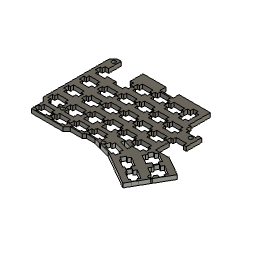
open-backplate-heatset-insert (Autodesk Fusion 360 design; units mm, degrees)
Autodesk Fusion 360 part; units mm, degrees
sketch "Sketch1" plane through (0, 0, 0) normal (0, 0, 1) x (1, 0, 0)
  line L0 (38.6885, 37.314) -> (36.2135, 37.314)
  line L1 (36.2135, 37.314) -> (36.2135, 63.246)
  line L2 (36.2135, 63.246) -> (-1.4615, 63.246)
  line L3 (-1.4615, 63.246) -> (-1.4615, 56.246)
  line L4 (-1.4615, 56.246) -> (-17.4615, 56.246)
  line L5 (-17.4615, 56.246) -> (-17.4615, 63.246)
  line L6 (-17.4615, 63.246) -> (-45.1095, 63.246)
  line L7 (-45.1095, 63.246) -> (-45.1095, 47.839)
  line L8 (-45.1095, 47.839) -> (-41.2315, 47.839)
  line L9 (-41.2315, 47.839) -> (-41.2315, 44.299)
  line L10 (-41.2315, 44.299) -> (-38.5615, 44.299)
  line L11 (-38.5615, 44.299) -> (-38.5615, 38.759)
  line L12 (-38.5615, 38.759) -> (-42.0615, 38.759)
  line L13 (-42.0615, 38.759) -> (-42.0615, 35.339)
  line L14 (-42.0615, 35.339) -> (-53.0615, 35.339)
  line L15 (-53.0615, 35.339) -> (-53.0615, 38.759)
  line L16 (-53.0615, 38.759) -> (-63.6515, 38.759)
  line L17 (-63.6515, 38.759) -> (-63.6515, 35.339)
  line L18 (-63.6515, 35.339) -> (-74.6515, 35.339)
  line L19 (-74.6515, 35.339) -> (-74.6515, 38.759)
  line L20 (-74.6515, 38.759) -> (-78.1515, 38.759)
  line L21 (-78.1515, 38.759) -> (-78.1515, 44.299)
  line L22 (-78.1515, 44.299) -> (-75.4815, 44.299)
  line L23 (-75.4815, 44.299) -> (-75.4815, 47.839)
  line L24 (-75.4815, 47.839) -> (-71.3495, 47.839)
  line L25 (-71.3495, 47.839) -> (-71.3495, 63.246)
  line L26 (-71.3495, 63.246) -> (-76.0095, 63.246)
  line L27 (-76.0095, 63.246) -> (-81.0895, 58.166)
  line L28 (-81.0895, 58.166) -> (-81.0895, -21.336)
  line L29 (-81.0895, -21.336) -> (-76.2635, -26.162)
  line L30 (-76.2635, -26.162) -> (-76.2635, -40.386)
  line L31 (-76.2635, -40.386) -> (-38.1635, -40.386)
  line L32 (-38.1635, -40.386) -> (-33.8455, -36.068)
  line L33 (-33.8455, -36.068) -> (-19.1135, -36.068)
  line L34 (-19.1135, -36.068) -> (-16.5735, -33.528)
  line L35 (-16.5735, -33.528) -> (-6.4135, -33.528)
  line L36 (-6.4135, -33.528) -> (1.2965, -35.5781)
  line L37 (1.2965, -35.5781) -> (0.5808, -35.056)
  line L38 (0.5808, -35.056) -> (0.019, -34.371)
  line L39 (0.019, -34.371) -> (-0.3528, -33.5668)
  line L40 (-0.3528, -33.5668) -> (-0.5107, -32.6951)
  line L41 (-0.5107, -32.6951) -> (-0.4447, -31.8116)
  line L42 (-0.4447, -31.8116) -> (-0.159, -30.973)
  line L43 (-0.159, -30.973) -> (0.3281, -30.233)
  line L44 (0.3281, -30.233) -> (0.9854, -29.6391)
  line L45 (0.9854, -29.6391) -> (1.7708, -29.2292)
  line L46 (1.7708, -29.2292) -> (2.634, -29.0296)
  line L47 (2.634, -29.0296) -> (3.5196, -29.0532)
  line L48 (3.5196, -29.0532) -> (4.3709, -29.2983)
  line L49 (4.3709, -29.2983) -> (5.1334, -29.7494)
  line L50 (5.1334, -29.7494) -> (5.7582, -30.3775)
  line L51 (5.7582, -30.3775) -> (6.2053, -31.1423)
  line L52 (6.2053, -31.1423) -> (6.976, -28.2662)
  line L53 (6.976, -28.2662) -> (9.555, -28.9572)
  line L54 (9.555, -28.9572) -> (10.4712, -25.5379)
  line L55 (10.4712, -25.5379) -> (22.6999, -28.8145)
  line L56 (22.6999, -28.8145) -> (21.7836, -32.2339)
  line L57 (21.7836, -32.2339) -> (24.3627, -32.9249)
  line L58 (24.3627, -32.9249) -> (22.9288, -38.2762)
  line L59 (22.9288, -38.2762) -> (19.5481, -37.3703)
  line L60 (19.5481, -37.3703) -> (19.1145, -38.9882)
  line L61 (19.1145, -38.9882) -> (8.4894, -36.1412)
  line L62 (8.4894, -36.1412) -> (8.9229, -34.5233)
  line L63 (8.9229, -34.5233) -> (6.2374, -33.8037)
  line L64 (6.2374, -33.8037) -> (5.8334, -34.5452)
  line L65 (5.8334, -34.5452) -> (5.2635, -35.1684)
  line L66 (5.2635, -35.1684) -> (4.5609, -35.6369)
  line L67 (4.5609, -35.6369) -> (3.7666, -35.9235)
  line L68 (3.7666, -35.9235) -> (2.9267, -36.0115)
  line L69 (2.9267, -36.0115) -> (15.5575, -39.37)
  line L70 (15.5575, -39.37) -> (56.9595, -63.246)
  line L71 (56.9595, -63.246) -> (57.0865, -63.246)
  line L72 (57.0865, -63.246) -> (69.3649, -41.9374)
  line L73 (69.3649, -41.9374) -> (68.7057, -42.5189)
  line L74 (68.7057, -42.5189) -> (67.9224, -42.9177)
  line L75 (67.9224, -42.9177) -> (67.0644, -43.1088)
  line L76 (67.0644, -43.1088) -> (66.1858, -43.0801)
  line L77 (66.1858, -43.0801) -> (65.3421, -42.8334)
  line L78 (65.3421, -42.8334) -> (64.5865, -42.3843)
  line L79 (64.5865, -42.3843) -> (63.9667, -41.761)
  line L80 (63.9667, -41.761) -> (63.5216, -41.003)
  line L81 (63.5216, -41.003) -> (63.2795, -40.158)
  line L82 (63.2795, -40.158) -> (63.2555, -39.2793)
  line L83 (63.2555, -39.2793) -> (63.4512, -38.4224)
  line L84 (63.4512, -38.4224) -> (63.8543, -37.6412)
  line L85 (63.8543, -37.6412) -> (64.4393, -36.9851)
  line L86 (64.4393, -36.9851) -> (56.2282, -32.2241)
  line L87 (56.2282, -32.2241) -> (57.7331, -29.6288)
  line L88 (57.7331, -29.6288) -> (58.953, -27.5158)
  line L89 (58.953, -27.5158) -> (56.9243, -26.3445)
  line L90 (56.9243, -26.3445) -> (59.6943, -21.5467)
  line L91 (59.6943, -21.5467) -> (62.0066, -22.8817)
  line L92 (62.0066, -22.8817) -> (63.7766, -19.8159)
  line L93 (63.7766, -19.8159) -> (74.7404, -26.1459)
  line L94 (74.7404, -26.1459) -> (72.9704, -29.2117)
  line L95 (72.9704, -29.2117) -> (75.2827, -30.5467)
  line L96 (75.2827, -30.5467) -> (72.5127, -35.3445)
  line L97 (72.5127, -35.3445) -> (69.7783, -33.7657)
  line L98 (69.7783, -33.7657) -> (68.5467, -35.8989)
  line L99 (68.5467, -35.8989) -> (68.2253, -36.4557)
  line L100 (68.2253, -36.4557) -> (68.9421, -36.9048)
  line L101 (68.9421, -36.9048) -> (69.5309, -37.5139)
  line L102 (69.5309, -37.5139) -> (69.956, -38.2466)
  line L103 (69.956, -38.2466) -> (70.1927, -39.0599)
  line L104 (70.1927, -39.0599) -> (70.2271, -39.9063)
  line L105 (70.2271, -39.9063) -> (70.0571, -40.7362)
  line L106 (70.0571, -40.7362) -> (81.0895, -21.59)
  line L107 (81.0895, -21.59) -> (57.2135, -7.874)
  line L108 (57.2135, -7.874) -> (57.2135, -8.776)
  line L109 (57.2135, -8.776) -> (42.1885, -8.776)
  line L110 (42.1885, -8.776) -> (42.1885, 7.644)
  line L111 (42.1885, 7.644) -> (38.6885, 7.644)
  line L112 (38.6885, 7.644) -> (38.6885, 13.184)
  line L113 (38.6885, 13.184) -> (41.3585, 13.184)
  line L114 (41.3585, 13.184) -> (41.3585, 16.724)
  line L115 (41.3585, 16.724) -> (54.0185, 16.724)
  line L116 (54.0185, 16.724) -> (54.0185, 13.184)
  line L117 (54.0185, 13.184) -> (57.2135, 13.184)
  line L118 (57.2135, 13.184) -> (57.2135, 31.774)
  line L119 (57.2135, 31.774) -> (53.1885, 31.774)
  line L120 (53.1885, 31.774) -> (53.1885, 28.354)
  line L121 (53.1885, 28.354) -> (52.1361, 28.354)
  line L122 (52.1361, 28.354) -> (52.9138, 27.8863)
  line L123 (52.9138, 27.8863) -> (53.5451, 27.2344)
  line L124 (53.5451, 27.2344) -> (53.9877, 26.4421)
  line L125 (53.9877, 26.4421) -> (54.2116, 25.5627)
  line L126 (54.2116, 25.5627) -> (54.2019, 24.6552)
  line L127 (54.2019, 24.6552) -> (53.9593, 23.7808)
  line L128 (53.9593, 23.7808) -> (53.4999, 22.9981)
  line L129 (53.4999, 22.9981) -> (52.8548, 22.3598)
  line L130 (52.8548, 22.3598) -> (52.0673, 21.9089)
  line L131 (52.0673, 21.9089) -> (51.1903, 21.6755)
  line L132 (51.1903, 21.6755) -> (50.2828, 21.6755)
  line L133 (50.2828, 21.6755) -> (49.4057, 21.9089)
  line L134 (49.4057, 21.9089) -> (48.6182, 22.3598)
  line L135 (48.6182, 22.3598) -> (47.9731, 22.9981)
  line L136 (47.9731, 22.9981) -> (47.5137, 23.7808)
  line L137 (47.5137, 23.7808) -> (47.2711, 24.6552)
  line L138 (47.2711, 24.6552) -> (47.2614, 25.5627)
  line L139 (47.2614, 25.5627) -> (47.4853, 26.4421)
  line L140 (47.4853, 26.4421) -> (47.9279, 27.2344)
  line L141 (47.9279, 27.2344) -> (48.5592, 27.8863)
  line L142 (48.5592, 27.8863) -> (49.337, 28.354)
  line L143 (49.337, 28.354) -> (42.1885, 28.354)
  line L144 (42.1885, 28.354) -> (42.1885, 31.774)
  line L145 (42.1885, 31.774) -> (38.6885, 31.774)
  line L146 (38.6885, 31.774) -> (38.6885, 37.314)
  line L147 (-71.8668, 59.0719) -> (-71.7475, 58.166)
  line L148 (-71.7475, 58.166) -> (-71.8668, 57.2601)
  line L149 (-71.8668, 57.2601) -> (-72.2164, 56.416)
  line L150 (-72.2164, 56.416) -> (-72.7726, 55.6911)
  line L151 (-72.7726, 55.6911) -> (-73.4975, 55.1349)
  line L152 (-73.4975, 55.1349) -> (-74.3416, 54.7853)
  line L153 (-74.3416, 54.7853) -> (-75.2475, 54.666)
  line L154 (-75.2475, 54.666) -> (-76.1534, 54.7853)
  line L155 (-76.1534, 54.7853) -> (-76.9975, 55.1349)
  line L156 (-76.9975, 55.1349) -> (-77.7224, 55.6911)
  line L157 (-77.7224, 55.6911) -> (-78.2786, 56.416)
  line L158 (-78.2786, 56.416) -> (-78.6282, 57.2601)
  line L159 (-78.6282, 57.2601) -> (-78.7475, 58.166)
  line L160 (-78.7475, 58.166) -> (-78.6282, 59.0719)
  line L161 (-78.6282, 59.0719) -> (-78.2786, 59.916)
  line L162 (-78.2786, 59.916) -> (-77.7224, 60.6409)
  line L163 (-77.7224, 60.6409) -> (-76.9975, 61.1971)
  line L164 (-76.9975, 61.1971) -> (-76.1534, 61.5467)
  line L165 (-76.1534, 61.5467) -> (-75.2475, 61.666)
  line L166 (-75.2475, 61.666) -> (-74.3416, 61.5467)
  line L167 (-74.3416, 61.5467) -> (-73.4975, 61.1971)
  line L168 (-73.4975, 61.1971) -> (-72.7726, 60.6409)
  line L169 (-72.7726, 60.6409) -> (-72.2164, 59.916)
  line L170 (-72.2164, 59.916) -> (-71.8668, 59.0719)
  line L171 (-53.0615, -18.4285) -> (-55.7119, -18.4285)
  line L172 (-55.7119, -18.4285) -> (-54.9733, -18.9008)
  line L173 (-54.9733, -18.9008) -> (-54.3753, -19.5419)
  line L174 (-54.3753, -19.5419) -> (-53.9554, -20.3114)
  line L175 (-53.9554, -20.3114) -> (-53.7399, -21.1611)
  line L176 (-53.7399, -21.1611) -> (-53.7423, -22.0378)
  line L177 (-53.7423, -22.0378) -> (-53.9624, -22.8863)
  line L178 (-53.9624, -22.8863) -> (-54.3865, -23.6536)
  line L179 (-54.3865, -23.6536) -> (-54.988, -24.2913)
  line L180 (-54.988, -24.2913) -> (-55.7291, -24.7596)
  line L181 (-55.7291, -24.7596) -> (-56.5633, -25.0291)
  line L182 (-56.5633, -25.0291) -> (-57.4383, -25.0828)
  line L183 (-57.4383, -25.0828) -> (-58.2992, -24.9174)
  line L184 (-58.2992, -24.9174) -> (-59.092, -24.5432)
  line L185 (-59.092, -24.5432) -> (-59.7669, -23.9837)
  line L186 (-59.7669, -23.9837) -> (-60.2817, -23.2741)
  line L187 (-60.2817, -23.2741) -> (-60.6039, -22.4589)
  line L188 (-60.6039, -22.4589) -> (-60.7135, -21.5891)
  line L189 (-60.7135, -21.5891) -> (-60.6035, -20.7194)
  line L190 (-60.6035, -20.7194) -> (-60.2808, -19.9043)
  line L191 (-60.2808, -19.9043) -> (-59.7657, -19.1949)
  line L192 (-59.7657, -19.1949) -> (-59.0904, -18.6358)
  line L193 (-59.0904, -18.6358) -> (-58.2975, -18.2621)
  line L194 (-58.2975, -18.2621) -> (-57.4365, -18.0971)
  line L195 (-57.4365, -18.0971) -> (-56.5615, -18.1513)
  line L196 (-56.5615, -18.1513) -> (-56.5615, -12.8885)
  line L197 (-56.5615, -12.8885) -> (-53.8915, -12.8885)
  line L198 (-53.8915, -12.8885) -> (-53.8915, -9.3485)
  line L199 (-53.8915, -9.3485) -> (-41.2315, -9.3485)
  line L200 (-41.2315, -9.3485) -> (-41.2315, -12.8885)
  line L201 (-41.2315, -12.8885) -> (-38.5615, -12.8885)
  line L202 (-38.5615, -12.8885) -> (-38.5615, -18.4285)
  line L203 (-38.5615, -18.4285) -> (-42.0615, -18.4285)
  line L204 (-42.0615, -18.4285) -> (-42.0615, -23.852)
  line L205 (-42.0615, -23.852) -> (-53.0615, -23.852)
  line L206 (-53.0615, -23.852) -> (-53.0615, -18.4285)
  line L207 (-53.0615, -37.491) -> (-53.0615, -39.166)
  line L208 (-53.0615, -39.166) -> (-42.0615, -39.166)
  line L209 (-42.0615, -39.166) -> (-42.0615, -37.491)
  line L210 (-42.0615, -37.491) -> (-38.5615, -37.491)
  line L211 (-38.5615, -37.491) -> (-38.5615, -31.951)
  line L212 (-38.5615, -31.951) -> (-41.2315, -31.951)
  line L213 (-41.2315, -31.951) -> (-41.2315, -28.411)
  line L214 (-41.2315, -28.411) -> (-53.8915, -28.411)
  line L215 (-53.8915, -28.411) -> (-53.8915, -31.951)
  line L216 (-53.8915, -31.951) -> (-56.5615, -31.951)
  line L217 (-56.5615, -31.951) -> (-56.5615, -37.491)
  line L218 (-56.5615, -37.491) -> (-53.0615, -37.491)
  line L219 (-14.9615, -30.506) -> (-14.9615, -32.181)
  line L220 (-14.9615, -32.181) -> (-3.9615, -32.181)
  line L221 (-3.9615, -32.181) -> (-3.9615, -30.506)
  line L222 (-3.9615, -30.506) -> (-0.4615, -30.506)
  line L223 (-0.4615, -30.506) -> (-0.4615, -24.966)
  line L224 (-0.4615, -24.966) -> (-3.1315, -24.966)
  line L225 (-3.1315, -24.966) -> (-3.1315, -21.426)
  line L226 (-3.1315, -21.426) -> (-15.7915, -21.426)
  line L227 (-15.7915, -21.426) -> (-15.7915, -24.966)
  line L228 (-15.7915, -24.966) -> (-18.4615, -24.966)
  line L229 (-18.4615, -24.966) -> (-18.4615, -30.506)
  line L230 (-18.4615, -30.506) -> (-14.9615, -30.506)
  line L231 (47.8904, -49.0495) -> (47.0529, -50.5)
  line L232 (47.0529, -50.5) -> (56.5791, -56)
  line L233 (56.5791, -56) -> (57.4166, -54.5495)
  line L234 (57.4166, -54.5495) -> (60.4477, -56.2995)
  line L235 (60.4477, -56.2995) -> (63.2177, -51.5017)
  line L236 (63.2177, -51.5017) -> (60.9054, -50.1667)
  line L237 (60.9054, -50.1667) -> (62.6754, -47.1009)
  line L238 (62.6754, -47.1009) -> (51.7116, -40.7709)
  line L239 (51.7116, -40.7709) -> (49.9416, -43.8367)
  line L240 (49.9416, -43.8367) -> (47.6293, -42.5017)
  line L241 (47.6293, -42.5017) -> (44.8593, -47.2995)
  line L242 (44.8593, -47.2995) -> (47.8904, -49.0495)
  line L243 (31.3804, -39.5245) -> (30.5429, -40.9751)
  line L244 (30.5429, -40.9751) -> (40.0691, -46.4751)
  line L245 (40.0691, -46.4751) -> (40.9066, -45.0245)
  line L246 (40.9066, -45.0245) -> (43.9377, -46.7745)
  line L247 (43.9377, -46.7745) -> (46.7077, -41.9767)
  line L248 (46.7077, -41.9767) -> (44.3954, -40.6417)
  line L249 (44.3954, -40.6417) -> (46.1654, -37.5759)
  line L250 (46.1654, -37.5759) -> (35.2016, -31.2459)
  line L251 (35.2016, -31.2459) -> (33.4316, -34.3117)
  line L252 (33.4316, -34.3117) -> (31.1193, -32.9767)
  line L253 (31.1193, -32.9767) -> (28.3493, -37.7745)
  line L254 (28.3493, -37.7745) -> (31.3804, -39.5245)
  line L255 (-72.1115, -37.441) -> (-72.1115, -39.1189)
  line L256 (-72.1115, -39.1189) -> (-61.1115, -39.1189)
  line L257 (-61.1115, -39.1189) -> (-61.1115, -37.441)
  line L258 (-61.1115, -37.441) -> (-57.6115, -37.441)
  line L259 (-57.6115, -37.441) -> (-57.6115, -31.901)
  line L260 (-57.6115, -31.901) -> (-60.2815, -31.901)
  line L261 (-60.2815, -31.901) -> (-60.2815, -28.361)
  line L262 (-60.2815, -28.361) -> (-72.9415, -28.361)
  line L263 (-72.9415, -28.361) -> (-72.9415, -31.901)
  line L264 (-72.9415, -31.901) -> (-75.6115, -31.901)
  line L265 (-75.6115, -31.901) -> (-75.6115, -37.441)
  line L266 (-75.6115, -37.441) -> (-72.1115, -37.441)
  line L267 (-0.4615, 7.619) -> (-0.4615, 13.159)
  line L268 (-0.4615, 13.159) -> (-3.1315, 13.159)
  line L269 (-3.1315, 13.159) -> (-3.1315, 16.699)
  line L270 (-3.1315, 16.699) -> (-15.7915, 16.699)
  line L271 (-15.7915, 16.699) -> (-15.7915, 13.159)
  line L272 (-15.7915, 13.159) -> (-18.4615, 13.159)
  line L273 (-18.4615, 13.159) -> (-18.4615, 7.619)
  line L274 (-18.4615, 7.619) -> (-14.9615, 7.619)
  line L275 (-14.9615, 7.619) -> (-14.9615, 4.199)
  line L276 (-14.9615, 4.199) -> (-3.9615, 4.199)
  line L277 (-3.9615, 4.199) -> (-3.9615, 7.619)
  line L278 (-3.9615, 7.619) -> (-0.4615, 7.619)
  line L279 (-34.0115, -33.046) -> (-34.0115, -34.721)
  line L280 (-34.0115, -34.721) -> (-23.0115, -34.721)
  line L281 (-23.0115, -34.721) -> (-23.0115, -33.046)
  line L282 (-23.0115, -33.046) -> (-19.5115, -33.046)
  line L283 (-19.5115, -33.046) -> (-19.5115, -27.506)
  line L284 (-19.5115, -27.506) -> (-22.1815, -27.506)
  line L285 (-22.1815, -27.506) -> (-22.1815, -23.966)
  line L286 (-22.1815, -23.966) -> (-34.8415, -23.966)
  line L287 (-34.8415, -23.966) -> (-34.8415, -27.506)
  line L288 (-34.8415, -27.506) -> (-37.5115, -27.506)
  line L289 (-37.5115, -27.506) -> (-37.5115, -33.046)
  line L290 (-37.5115, -33.046) -> (-34.0115, -33.046)
  line L291 (-19.5115, 43.204) -> (-19.5115, 48.744)
  line L292 (-19.5115, 48.744) -> (-22.1815, 48.744)
  line L293 (-22.1815, 48.744) -> (-22.1815, 52.284)
  line L294 (-22.1815, 52.284) -> (-34.8415, 52.284)
  line L295 (-34.8415, 52.284) -> (-34.8415, 48.744)
  line L296 (-34.8415, 48.744) -> (-37.5115, 48.744)
  line L297 (-37.5115, 48.744) -> (-37.5115, 43.204)
  line L298 (-37.5115, 43.204) -> (-34.0115, 43.204)
  line L299 (-34.0115, 43.204) -> (-34.0115, 39.784)
  line L300 (-34.0115, 39.784) -> (-23.0115, 39.784)
  line L301 (-23.0115, 39.784) -> (-23.0115, 43.204)
  line L302 (-23.0115, 43.204) -> (-19.5115, 43.204)
  line L303 (15.9185, -8.256) -> (15.9185, -4.716)
  line L304 (15.9185, -4.716) -> (3.2585, -4.716)
  line L305 (3.2585, -4.716) -> (3.2585, -8.256)
  line L306 (3.2585, -8.256) -> (0.5885, -8.256)
  line L307 (0.5885, -8.256) -> (0.5885, -13.796)
  line L308 (0.5885, -13.796) -> (4.0885, -13.796)
  line L309 (4.0885, -13.796) -> (4.0885, -17.216)
  line L310 (4.0885, -17.216) -> (15.0885, -17.216)
  line L311 (15.0885, -17.216) -> (15.0885, -13.796)
  line L312 (15.0885, -13.796) -> (18.5885, -13.796)
  line L313 (18.5885, -13.796) -> (18.5885, -8.256)
  line L314 (18.5885, -8.256) -> (15.9185, -8.256)
  line L315 (-34.0115, -13.9835) -> (-34.0115, -19.534)
  line L316 (-34.0115, -19.534) -> (-23.0115, -19.534)
  line L317 (-23.0115, -19.534) -> (-23.0115, -13.9835)
  line L318 (-23.0115, -13.9835) -> (-19.5115, -13.9835)
  line L319 (-19.5115, -13.9835) -> (-19.5115, -8.4435)
  line L320 (-19.5115, -8.4435) -> (-22.1815, -8.4435)
  line L321 (-22.1815, -8.4435) -> (-22.1815, -4.9035)
  line L322 (-22.1815, -4.9035) -> (-34.8415, -4.9035)
  line L323 (-34.8415, -4.9035) -> (-34.8415, -8.4435)
  line L324 (-34.8415, -8.4435) -> (-37.5115, -8.4435)
  line L325 (-37.5115, -8.4435) -> (-37.5115, -13.9835)
  line L326 (-37.5115, -13.9835) -> (-34.0115, -13.9835)
  line L327 (58.7727, -21.0217) -> (56.4604, -19.6867)
  line L328 (56.4604, -19.6867) -> (58.2304, -16.6209)
  line L329 (58.2304, -16.6209) -> (47.2666, -10.2909)
  line L330 (47.2666, -10.2909) -> (45.4966, -13.3567)
  line L331 (45.4966, -13.3567) -> (43.1843, -12.0217)
  line L332 (43.1843, -12.0217) -> (40.4143, -16.8195)
  line L333 (40.4143, -16.8195) -> (42.443, -17.9908)
  line L334 (42.443, -17.9908) -> (41.2231, -20.1038)
  line L335 (41.2231, -20.1038) -> (39.7182, -22.6991)
  line L336 (39.7182, -22.6991) -> (50.5319, -28.9692)
  line L337 (50.5319, -28.9692) -> (52.0367, -26.3739)
  line L338 (52.0367, -26.3739) -> (53.2683, -24.2408)
  line L339 (53.2683, -24.2408) -> (56.0027, -25.8195)
  line L340 (56.0027, -25.8195) -> (58.7727, -21.0217)
  line L341 (-19.5115, 10.619) -> (-22.1815, 10.619)
  line L342 (-22.1815, 10.619) -> (-22.1815, 14.159)
  line L343 (-22.1815, 14.159) -> (-34.8415, 14.159)
  line L344 (-34.8415, 14.159) -> (-34.8415, 10.619)
  line L345 (-34.8415, 10.619) -> (-37.5115, 10.619)
  line L346 (-37.5115, 10.619) -> (-37.5115, 5.079)
  line L347 (-37.5115, 5.079) -> (-34.0115, 5.079)
  line L348 (-34.0115, 5.079) -> (-34.0115, 1.659)
  line L349 (-34.0115, 1.659) -> (-23.0115, 1.659)
  line L350 (-23.0115, 1.659) -> (-23.0115, 5.079)
  line L351 (-23.0115, 5.079) -> (-19.5115, 5.079)
  line L352 (-19.5115, 5.079) -> (-19.5115, 10.619)
  line L353 (15.9185, 10.744) -> (15.9185, 14.284)
  line L354 (15.9185, 14.284) -> (3.2585, 14.284)
  line L355 (3.2585, 14.284) -> (3.2585, 10.744)
  line L356 (3.2585, 10.744) -> (0.5885, 10.744)
  line L357 (0.5885, 10.744) -> (0.5885, 5.204)
  line L358 (0.5885, 5.204) -> (4.0885, 5.204)
  line L359 (4.0885, 5.204) -> (4.0885, 1.784)
  line L360 (4.0885, 1.784) -> (15.0885, 1.784)
  line L361 (15.0885, 1.784) -> (15.0885, 5.204)
  line L362 (15.0885, 5.204) -> (18.5885, 5.204)
  line L363 (18.5885, 5.204) -> (18.5885, 10.744)
  line L364 (18.5885, 10.744) -> (15.9185, 10.744)
  line L365 (22.0585, 38.879) -> (27.5985, 38.879)
  line L366 (27.5985, 38.879) -> (27.5985, 41.549)
  line L367 (27.5985, 41.549) -> (31.1385, 41.549)
  line L368 (31.1385, 41.549) -> (31.1385, 54.209)
  line L369 (31.1385, 54.209) -> (27.5985, 54.209)
  line L370 (27.5985, 54.209) -> (27.5985, 56.879)
  line L371 (27.5985, 56.879) -> (22.0585, 56.879)
  line L372 (22.0585, 56.879) -> (22.0585, 53.379)
  line L373 (22.0585, 53.379) -> (18.6385, 53.379)
  line L374 (18.6385, 53.379) -> (18.6385, 42.379)
  line L375 (18.6385, 42.379) -> (22.0585, 42.379)
  line L376 (22.0585, 42.379) -> (22.0585, 38.879)
  line L377 (23.1385, 22.249) -> (23.1385, 18.829)
  line L378 (23.1385, 18.829) -> (34.1385, 18.829)
  line L379 (34.1385, 18.829) -> (34.1385, 22.249)
  line L380 (34.1385, 22.249) -> (37.6385, 22.249)
  line L381 (37.6385, 22.249) -> (37.6385, 27.789)
  line L382 (37.6385, 27.789) -> (34.9685, 27.789)
  line L383 (34.9685, 27.789) -> (34.9685, 31.329)
  line L384 (34.9685, 31.329) -> (22.3085, 31.329)
  line L385 (22.3085, 31.329) -> (22.3085, 27.789)
  line L386 (22.3085, 27.789) -> (19.6385, 27.789)
  line L387 (19.6385, 27.789) -> (19.6385, 22.249)
  line L388 (19.6385, 22.249) -> (23.1385, 22.249)
  line L389 (-0.4615, 26.6815) -> (-0.4615, 32.2215)
  line L390 (-0.4615, 32.2215) -> (-3.1315, 32.2215)
  line L391 (-3.1315, 32.2215) -> (-3.1315, 35.7615)
  line L392 (-3.1315, 35.7615) -> (-15.7915, 35.7615)
  line L393 (-15.7915, 35.7615) -> (-15.7915, 32.2215)
  line L394 (-15.7915, 32.2215) -> (-18.4615, 32.2215)
  line L395 (-18.4615, 32.2215) -> (-18.4615, 26.6815)
  line L396 (-18.4615, 26.6815) -> (-14.9615, 26.6815)
  line L397 (-14.9615, 26.6815) -> (-14.9615, 23.2615)
  line L398 (-14.9615, 23.2615) -> (-3.9615, 23.2615)
  line L399 (-3.9615, 23.2615) -> (-3.9615, 26.6815)
  line L400 (-3.9615, 26.6815) -> (-0.4615, 26.6815)
  line L401 (-19.5115, 29.6815) -> (-22.1815, 29.6815)
  line L402 (-22.1815, 29.6815) -> (-22.1815, 33.2215)
  line L403 (-22.1815, 33.2215) -> (-34.8415, 33.2215)
  line L404 (-34.8415, 33.2215) -> (-34.8415, 29.6815)
  line L405 (-34.8415, 29.6815) -> (-37.5115, 29.6815)
  line L406 (-37.5115, 29.6815) -> (-37.5115, 24.1415)
  line L407 (-37.5115, 24.1415) -> (-34.0115, 24.1415)
  line L408 (-34.0115, 24.1415) -> (-34.0115, 20.7215)
  line L409 (-34.0115, 20.7215) -> (-23.0115, 20.7215)
  line L410 (-23.0115, 20.7215) -> (-23.0115, 24.1415)
  line L411 (-23.0115, 24.1415) -> (-19.5115, 24.1415)
  line L412 (-19.5115, 24.1415) -> (-19.5115, 29.6815)
  line L413 (-60.1515, 25.2157) -> (-62.8215, 25.2157)
  line L414 (-62.8215, 25.2157) -> (-62.8215, 28.7557)
  line L415 (-62.8215, 28.7557) -> (-75.4815, 28.7557)
  line L416 (-75.4815, 28.7557) -> (-75.4815, 25.2157)
  line L417 (-75.4815, 25.2157) -> (-78.1515, 25.2157)
  line L418 (-78.1515, 25.2157) -> (-78.1515, 19.6757)
  line L419 (-78.1515, 19.6757) -> (-74.6515, 19.6757)
  line L420 (-74.6515, 19.6757) -> (-74.6515, 16.2557)
  line L421 (-74.6515, 16.2557) -> (-63.6515, 16.2557)
  line L422 (-63.6515, 16.2557) -> (-63.6515, 19.6757)
  line L423 (-63.6515, 19.6757) -> (-60.1515, 19.6757)
  line L424 (-60.1515, 19.6757) -> (-60.1515, 25.2157)
  line L425 (15.9185, 29.744) -> (15.9185, 33.284)
  line L426 (15.9185, 33.284) -> (3.2585, 33.284)
  line L427 (3.2585, 33.284) -> (3.2585, 29.744)
  line L428 (3.2585, 29.744) -> (0.5885, 29.744)
  line L429 (0.5885, 29.744) -> (0.5885, 24.204)
  line L430 (0.5885, 24.204) -> (4.0885, 24.204)
  line L431 (4.0885, 24.204) -> (4.0885, 20.784)
  line L432 (4.0885, 20.784) -> (15.0885, 20.784)
  line L433 (15.0885, 20.784) -> (15.0885, 24.204)
  line L434 (15.0885, 24.204) -> (18.5885, 24.204)
  line L435 (18.5885, 24.204) -> (18.5885, 29.744)
  line L436 (18.5885, 29.744) -> (15.9185, 29.744)
  line L437 (18.5885, 48.744) -> (15.9185, 48.744)
  line L438 (15.9185, 48.744) -> (15.9185, 52.284)
  line L439 (15.9185, 52.284) -> (3.2585, 52.284)
  line L440 (3.2585, 52.284) -> (3.2585, 48.744)
  line L441 (3.2585, 48.744) -> (0.5885, 48.744)
  line L442 (0.5885, 48.744) -> (0.5885, 43.204)
  line L443 (0.5885, 43.204) -> (4.0885, 43.204)
  line L444 (4.0885, 43.204) -> (4.0885, 39.784)
  line L445 (4.0885, 39.784) -> (15.0885, 39.784)
  line L446 (15.0885, 39.784) -> (15.0885, 43.204)
  line L447 (15.0885, 43.204) -> (18.5885, 43.204)
  line L448 (18.5885, 43.204) -> (18.5885, 48.744)
  line L449 (34.9685, 8.789) -> (34.9685, 12.329)
  line L450 (34.9685, 12.329) -> (22.3085, 12.329)
  line L451 (22.3085, 12.329) -> (22.3085, 8.789)
  line L452 (22.3085, 8.789) -> (19.6385, 8.789)
  line L453 (19.6385, 8.789) -> (19.6385, 3.249)
  line L454 (19.6385, 3.249) -> (23.1385, 3.249)
  line L455 (23.1385, 3.249) -> (23.1385, -0.171)
  line L456 (23.1385, -0.171) -> (34.1385, -0.171)
  line L457 (34.1385, -0.171) -> (34.1385, 3.249)
  line L458 (34.1385, 3.249) -> (37.6385, 3.249)
  line L459 (37.6385, 3.249) -> (37.6385, 8.789)
  line L460 (37.6385, 8.789) -> (34.9685, 8.789)
  line L461 (-53.0615, 19.6965) -> (-53.0615, 16.2765)
  line L462 (-53.0615, 16.2765) -> (-42.0615, 16.2765)
  line L463 (-42.0615, 16.2765) -> (-42.0615, 19.6965)
  line L464 (-42.0615, 19.6965) -> (-38.5615, 19.6965)
  line L465 (-38.5615, 19.6965) -> (-38.5615, 25.2365)
  line L466 (-38.5615, 25.2365) -> (-41.2315, 25.2365)
  line L467 (-41.2315, 25.2365) -> (-41.2315, 28.7765)
  line L468 (-41.2315, 28.7765) -> (-53.8915, 28.7765)
  line L469 (-53.8915, 28.7765) -> (-53.8915, 25.2365)
  line L470 (-53.8915, 25.2365) -> (-56.5615, 25.2365)
  line L471 (-56.5615, 25.2365) -> (-56.5615, 19.6965)
  line L472 (-56.5615, 19.6965) -> (-53.0615, 19.6965)
  line L473 (-14.9615, -11.4435) -> (-14.9615, -16.994)
  line L474 (-14.9615, -16.994) -> (-3.9615, -16.994)
  line L475 (-3.9615, -16.994) -> (-3.9615, -11.4435)
  line L476 (-3.9615, -11.4435) -> (-0.4615, -11.4435)
  line L477 (-0.4615, -11.4435) -> (-0.4615, -5.9035)
  line L478 (-0.4615, -5.9035) -> (-3.1315, -5.9035)
  line L479 (-3.1315, -5.9035) -> (-3.1315, -2.3635)
  line L480 (-3.1315, -2.3635) -> (-15.7915, -2.3635)
  line L481 (-15.7915, -2.3635) -> (-15.7915, -5.9035)
  line L482 (-15.7915, -5.9035) -> (-18.4615, -5.9035)
  line L483 (-18.4615, -5.9035) -> (-18.4615, -11.4435)
  line L484 (-18.4615, -11.4435) -> (-14.9615, -11.4435)
  line L485 (-60.1515, 6.1323) -> (-62.8215, 6.1323)
  line L486 (-62.8215, 6.1323) -> (-62.8215, 9.6723)
  line L487 (-62.8215, 9.6723) -> (-75.4815, 9.6723)
  line L488 (-75.4815, 9.6723) -> (-75.4815, 6.1323)
  line L489 (-75.4815, 6.1323) -> (-78.1515, 6.1323)
  line L490 (-78.1515, 6.1323) -> (-78.1515, 0.5923)
  line L491 (-78.1515, 0.5923) -> (-74.6515, 0.5923)
  line L492 (-74.6515, 0.5923) -> (-74.6515, -2.8277)
  line L493 (-74.6515, -2.8277) -> (-63.6515, -2.8277)
  line L494 (-63.6515, -2.8277) -> (-63.6515, 0.5923)
  line L495 (-63.6515, 0.5923) -> (-60.1515, 0.5923)
  line L496 (-60.1515, 0.5923) -> (-60.1515, 6.1323)
  line L497 (-14.9615, 45.744) -> (-14.9615, 42.324)
  line L498 (-14.9615, 42.324) -> (-3.9615, 42.324)
  line L499 (-3.9615, 42.324) -> (-3.9615, 45.744)
  line L500 (-3.9615, 45.744) -> (-0.4615, 45.744)
  line L501 (-0.4615, 45.744) -> (-0.4615, 51.284)
  line L502 (-0.4615, 51.284) -> (-3.1315, 51.284)
  line L503 (-3.1315, 51.284) -> (-3.1315, 54.824)
  line L504 (-3.1315, 54.824) -> (-15.7915, 54.824)
  line L505 (-15.7915, 54.824) -> (-15.7915, 51.284)
  line L506 (-15.7915, 51.284) -> (-18.4615, 51.284)
  line L507 (-18.4615, 51.284) -> (-18.4615, 45.744)
  line L508 (-18.4615, 45.744) -> (-14.9615, 45.744)
  line L509 (34.9685, -10.211) -> (34.9685, -6.671)
  line L510 (34.9685, -6.671) -> (22.3085, -6.671)
  line L511 (22.3085, -6.671) -> (22.3085, -10.211)
  line L512 (22.3085, -10.211) -> (19.6385, -10.211)
  line L513 (19.6385, -10.211) -> (19.6385, -15.751)
  line L514 (19.6385, -15.751) -> (23.1385, -15.751)
  line L515 (23.1385, -15.751) -> (23.1385, -19.171)
  line L516 (23.1385, -19.171) -> (34.1385, -19.171)
  line L517 (34.1385, -19.171) -> (34.1385, -15.751)
  line L518 (34.1385, -15.751) -> (37.6385, -15.751)
  line L519 (37.6385, -15.751) -> (37.6385, -10.211)
  line L520 (37.6385, -10.211) -> (34.9685, -10.211)
  line L521 (-53.0615, 0.634) -> (-53.0615, -2.786)
  line L522 (-53.0615, -2.786) -> (-42.0615, -2.786)
  line L523 (-42.0615, -2.786) -> (-42.0615, 0.634)
  line L524 (-42.0615, 0.634) -> (-38.5615, 0.634)
  line L525 (-38.5615, 0.634) -> (-38.5615, 6.174)
  line L526 (-38.5615, 6.174) -> (-41.2315, 6.174)
  line L527 (-41.2315, 6.174) -> (-41.2315, 9.714)
  line L528 (-41.2315, 9.714) -> (-53.8915, 9.714)
  line L529 (-53.8915, 9.714) -> (-53.8915, 6.174)
  line L530 (-53.8915, 6.174) -> (-56.5615, 6.174)
  line L531 (-56.5615, 6.174) -> (-56.5615, 0.634)
  line L532 (-56.5615, 0.634) -> (-53.0615, 0.634)
  line L533 (-74.6515, -18.491) -> (-74.6515, -21.911)
  line L534 (-74.6515, -21.911) -> (-72.1115, -21.911)
  line L535 (-72.1115, -21.911) -> (-72.1115, -23.852)
  line L536 (-72.1115, -23.852) -> (-61.1115, -23.852)
  line L537 (-61.1115, -23.852) -> (-61.1115, -20.852)
  line L538 (-61.1115, -20.852) -> (-63.6515, -20.852)
  line L539 (-63.6515, -20.852) -> (-63.6515, -18.491)
  line L540 (-63.6515, -18.491) -> (-60.1515, -18.491)
  line L541 (-60.1515, -18.491) -> (-60.1515, -12.951)
  line L542 (-60.1515, -12.951) -> (-62.8215, -12.951)
  line L543 (-62.8215, -12.951) -> (-62.8215, -9.411)
  line L544 (-62.8215, -9.411) -> (-75.4815, -9.411)
  line L545 (-75.4815, -9.411) -> (-75.4815, -12.951)
  line L546 (-75.4815, -12.951) -> (-78.1515, -12.951)
  line L547 (-78.1515, -12.951) -> (-78.1515, -18.491)
  line L548 (-78.1515, -18.491) -> (-74.6515, -18.491)
  line L549 (13.8728, -18.2221) -> (12.967, -21.6029)
  line L550 (12.967, -21.6029) -> (23.5922, -24.4499)
  line L551 (23.5922, -24.4499) -> (24.498, -21.0691)
  line L552 (24.498, -21.0691) -> (13.8728, -18.2221)
  line L553 (6.2053, -31.1423) -> (5.5421, -33.6174)
  line L554 (5.5421, -33.6174) -> (6.2374, -33.8037)
  line L555 (1.2965, -35.5781) -> (2.9267, -36.0115)
  line L556 (70.0571, -40.7362) -> (69.3649, -41.9374)
  line L557 (68.2253, -36.4557) -> (67.0467, -38.497)
  line L558 (67.0467, -38.497) -> (64.4393, -36.9851)
  line L559 (49.337, 28.354) -> (52.1361, 28.354)
  circle A0 centre (-75.2475, 58.166) radius 2.3
  line L560 (-75.2475, 61.666) -> (-75.2475, 54.666)
  line L561 (-78.7475, 58.166) -> (-71.7475, 58.166)
  line L562 (47.2662, 25.109) -> (54.2068, 25.109)
  circle A1 centre (50.7365, 25.109) radius 2.3
  line L563 (66.7267, -39.6357) -> (66.1858, -43.0801)
  line L564 (66.7267, -39.6357) -> (70.2099, -39.4831)
  line L565 (66.7267, -39.6357) -> (63.2795, -40.158)
  circle A2 centre (66.7267, -39.6357) radius 2.3
  line L566 (2.634, -29.0296) -> (2.9845, -32.512)
  line L567 (2.9845, -32.512) -> (0.019, -34.371)
  line L568 (-0.4447, -31.8116) -> (2.9845, -32.512)
  line L569 (6.2053, -31.1423) -> (2.9845, -32.512)
  circle A3 centre (2.9845, -32.512) radius 2.3
  line L570 (-57.2135, -21.59) -> (-57.4365, -18.0971)
  line L571 (-57.2135, -21.59) -> (-60.6035, -20.7194)
  line L572 (-54.988, -24.2913) -> (-57.2135, -21.59)
  circle A4 centre (-57.2135, -21.59) radius 2.3
  line L573 (-56.5615, -18.1513) -> (-56.5615, -18.4285)
  line L574 (-55.7119, -18.4285) -> (-56.5615, -18.4285)
  point P0 (-75.2475, 58.166)
  point P1 (66.7267, -39.6357)
  point P2 (2.9845, -32.512)
  point P3 (-57.2135, -21.59)
  dimension "d1" = 4.6
  dimension "d2" = 4.6
  dimension "d4" = 4.6
  dimension "d5" = 4.6
  dimension "d6" = 4.6
  constraint collinear L52 L553
  constraint collinear L63 L554
  constraint collinear L98 L557
  constraint collinear L86 L558
  constraint parallel L121 L559
  constraint vertical L560
  constraint horizontal L561
  constraint midpoint L560 P0
  constraint coincident P0 A0.centre
  constraint midpoint L138 L562.start
  constraint midpoint L126 L562.end
  constraint horizontal L562
  constraint midpoint L562 A1.centre
  constraint coincident P1 L563.start
  constraint midpoint L104 L564.end
  constraint equal L564 L565
  constraint equal L563 L564
  constraint coincident P2 L566.end
  constraint equal L566 L569
  constraint equal L567 L568
  constraint coincident P3 L570.start
  constraint equal L570 L572
  constraint equal L570 L571
  constraint perpendicular L573 L574
  measures "d1" diameter of A0
  measures "d2" diameter of A1
  measures "d4" diameter of A2
  measures "d5" diameter of A3
  measures "d6" diameter of A4
extrude "Extrude1" add sketch "Sketch1" along normal blind 5 contours L0 L1 L2 L3 L4 L5 L6 L7 L8 L9 L10 L11 L12 L13 L14 L15 L16 L17 L18 L19 L20 L21 L22 L23 L24 L25 L26 L27 L28 L29 L30 L31 L32 L33 L34 L35 L36 L37 L38 L39 L40 L41 L42 L43 L44 L45 L46 L47 L48 L49 L50 L51 L52 L53 L54 L55 L56 L57 L58 L59 L60 L61 L62 L63 L64 L65 L66 L67 L68 L69 L70 L71 L72 L73 L74 L75 L76 L77 L78 L79 L80 L81 L82 L83 L84 L85 L86 L87 L88 L89 L90 L91 L92 L93 L94 L95 L96 L97 L98 L99 L100 L101 L102 L103 L104 L105 L106 L107 L108 L109 L110 L111 L112 L113 L114 L115 L116 L117 L118 L119 L120 L121 L122 L123 L124 L125 L126 L127 L128 L129 L130 L131 L132 L133 L134 L135 L136 L137 L138 L139 L140 L141 L142 L143 L144 L145 L146 | L122 L123 L124 L125 L126 L138 L139 L140 L141 L142 L559 L562 A1 | L126 L127 L128 L129 L130 L131 L132 L133 L134 L135 L136 L137 L138 L562 A1 | L562 A1 | L562 A1 | L73 L74 L75 L76 L104 L105 L556 L563 L564 A2 | L100 L101 L102 L103 L104 L557 L564 A2 | L563 L564 A2 | L557 L558 L564 L565 A2 | L563 L565 A2 | L77 L78 L79 L80 L81 L563 L565 A2 | L82 L83 L84 L85 L558 L565 A2 | L37 L38 L64 L65 L66 L67 L68 L553 L554 L555 L567 L569 A3 | L39 L40 L41 L567 L568 A3 | L567 L568 A3 | L567 L569 A3 | L566 L568 A3 | L566 L569 A3 | L42 L43 L44 L45 L46 L566 L568 A3 | L47 L48 L49 L50 L51 L566 L569 A3 | L147 L166 L167 L168 L169 L170 A0 L560 L561 | L148 L149 L150 L151 L152 L153 A0 L560 L561 | A0 L560 L561 | A0 L560 L561 | A0 L560 L561 | L160 L161 L162 L163 L164 L165 A0 L560 L561 | L154 L155 L156 L157 L158 L159 A0 L560 L561 | A0 L560 L561 | L172 L173 L174 L175 L176 L177 L178 L179 L195 L570 L572 A4 L573 L574 | L190 L191 L192 L193 L194 L570 L571 A4 | L570 L572 A4 | L570 L571 A4 | L571 L572 A4 | L180 L181 L182 L183 L184 L185 L186 L187 L188 L189 L571 L572 A4
extrude "Extrude2" cut sketch "Sketch1" along normal blind 3 from surface at 2 contours L562 A1 | L562 A1 | L563 L564 A2 | L557 L558 L564 L565 A2 | L563 L565 A2 | L557 L558 A2 | L567 L568 A3 | L567 L569 A3 | L566 L568 A3 | L566 L569 A3 | A0 L560 L561 | A0 L560 L561 | A0 L560 L561 | A0 L560 L561 | L570 L572 A4 | L570 L571 A4 | L571 L572 A4
equation "d1 = HoleSize"
equation "d2 = HoleSize"
equation "d4 = HoleSize"
equation "d5 = HoleSize"
equation "d6 = HoleSize"
equation "HoleSize = 4.6 mm"
